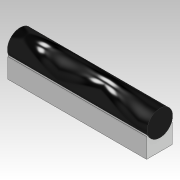
# Autodesk Inventor part: ApexSeal
Saved by Autodesk Inventor 2020 (Build 240168000, 168)
## iProperties
Created: 2021-10-16
Part Number: ApexSeal
Material: Generic
Document SubType Name: Modeling
Designer: DDeGo
Density: 1 g/cm^3
Appearance: Default
Author: DDeGo
Autodesk Inventor part; units mm, degrees
ref_plane "YZ Plane" through (0, 0, 0) normal (1, 0, 0) x (0, 1, 0)
ref_plane "XZ Plane" through (0, 0, 0) normal (0, 1, 0) x (-1, 0, 0)
ref_plane "XY Plane" through (0, 0, 0) normal (0, 0, 1) x (1, 0, 0)
sketch "Sketch1" plane through (0, 0, 0) normal (1, 0, 0) x (0, 1, 0)
  line L0 (-1, 1) -> (1, 1)
  line L1 (1, -1) -> (-1, -1)
  line L2 (-1, -1) -> (-1, 1)
  line L3 (-1, 1) -> (1, -1) construction
  line L4 (1, 1) -> (-1, -1) construction
  arc A0 (1, 1) -> (1, -1) centre (1, 0) ccw
  point P0 (0, 0)
  dimension "d0" = 2
  dimension "d1" = 2
  constraints: 10 end point, 2 midpoint, 2 point on circle, 2 tangent, 1 centre point, 1 horizontal, 1 parallel, 1 perpendicular
  measures "d0" distance between parallel lines of L1 L0
  measures "d1" distance of L1.start L1.end
extrude "Extrusion1" add sketch "Sketch1" along normal mid plane 10.9
fillet "Fillet1" radius 0.05 2 edges at (0, 1, 1) (0, 1, -1)
sketch "Sketch2" plane through (0, 0, 0) normal (1, 0, 0) x (0, 1, 0)
  arc A0 (1, 1) -> (1, -1) centre (1, 0) ccw projected
  circle A1 centre (1, 0) radius 1
  point P0 (0, 0)
  point P1 (1, 1)
  constraints: 1 coincident, 3 other
extrude "graphite" add sketch "Sketch2" along normal mid plane 11
body "Solid1"
